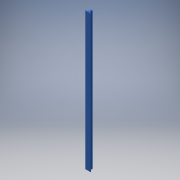
# Autodesk Inventor part: SBR16_EIXO_Y_2
Saved by Autodesk Inventor 2018 (Build 220112000, 112)
## iProperties
Created: 2018-10-09
Part Number: SBR16_EIXO_Y_2
Material: Genérico
Document SubType Name: Modeling
Designer: Georgines
Density: 1 g/cm^3
Appearance: Padrão
Author: Georgines
Autodesk Inventor part; units mm, degrees
ref_plane "YZ Plane" through (0, 0, 0) normal (1, 0, 0) x (0, 1, 0)
ref_plane "XZ Plane" through (0, 0, 0) normal (0, 1, 0) x (-1, 0, 0)
ref_plane "XY Plane" through (0, 0, 0) normal (0, 0, 1) x (1, 0, 0)
sketch "Esboço1" plane through (0, 0, 0) normal (0, 0, 1) x (1, 0, 0)
  arc A0 (4, 2.4377) -> (-4, 2.4377) centre (0, 9.3659) ccw
  line L0 (9.25, -3.9341) -> (9.25, -10.6341)
  line L1 (-9.25, -10.6341) -> (-9.25, -3.9341)
  line L2 (4, -15.6341) -> (-4, -15.6341)
  line L3 (20, -15.6341) -> (-20, -15.6341)
  line L4 (-20, -15.6341) -> (-20, -10.6341)
  line L5 (20, -10.6341) -> (20, -15.6341)
  line L6 (7.6788, -3.9341) -> (9.25, -3.9341)
  line L7 (-9.25, -3.9341) -> (-7.6788, -3.9341)
  line L8 (9.25, -10.6341) -> (20, -10.6341)
  line L9 (-20, -10.6341) -> (-9.25, -10.6341)
  line L10 (-4, 2.4377) -> (-7.6788, -3.9341)
  line L11 (-17.4151, -20.798) -> (-22.4188, -29.4646)
  line L12 (17.4151, -20.798) -> (23.6527, -31.6017)
  line L13 (9.25, -15.6341) -> (4, -15.6341)
  line L14 (0, -15.6341) -> (-9.25, -15.6341)
  line L15 (4, 2.4377) -> (7.6788, -3.9341)
  dimension "d6" = 16
  dimension "d7" = 25
  dimension "d8" = 18.5
  dimension "d9" = 11.7
  dimension "d10" = 8
  dimension "d13" = 5
  dimension "d14" = 40
  constraints: 32 end point, 8 parallel, 3 horizontal, 3 perpendicular, 2 point on circle, 1 centre point, 1 midpoint
  measures "d6" diameter of A0
  measures "d7" distance of A0.centre L14.start
  measures "d8" distance of L13.start L14.end
  measures "d9" distance of L0.start L13.start
  measures "d10" distance of L2.start L2.end
  measures "d13" distance of L3.end L4.end
  measures "d14" distance of L3.start L3.end
extrude "Extrusão1" add sketch "Esboço1" along normal blind 1054
sketch "Esboço3" plane through (-20, -15.6341, 0) normal (0, -1, 0) x (1, 0, 0)
  line L0 (0, 1054) -> (40, 1054) construction
  line L1 (20, 1054) -> (20, 0) construction
  line L2 (20, 1034) -> (5, 1034) construction
  line L3 (5, 1034) -> (20, 1034) construction
  line L4 (20, 1034) -> (35, 1034) construction
  circle A0 centre (5, 1034) radius 2.75
  circle A1 centre (35, 1034) radius 2.75
  line L5 (40, 0) -> (0, 0) construction
  dimension "d18" = 15
  dimension "d19" = 15
  dimension "d20" = 5.5
  dimension "d21" = 5.5
  dimension "d22" = 20
  constraints: 8 end point, 2 centre point, 2 coincident, 2 point on line, 1 collinear, 1 horizontal, 1 midpoint, 1 vertical
  measures "d18" distance of L2.start L2.end
  measures "d19" distance of L2.start L4.end
  measures "d20" diameter of A0
  measures "d21" diameter of A1
  measures "d22" distance between parallel lines of L0 L2
hole "Furo1" at (-15, -15.6341, 1034) at (15, -15.6341, 1034) direction (0, 1, 0) diameter 5.5 depth 8 tip angle 118
